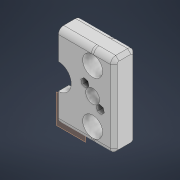
# Autodesk Inventor part: syringe_pump_sledge
Saved by Autodesk Inventor 2022 (Build 260153000, 153)
## iProperties
Created: 2023-04-03
Part Number: syringe_pump_sledge
Material: Generic
Document SubType Name: Modeling
Designer: Jakob Saugbjerg
Density: 1 g/cm^3
Appearance: Default
Author: Jakob Saugbjerg
Autodesk Inventor part; units mm, degrees
ref_plane "YZ Plane" through (0, 0, 0) normal (1, 0, 0) x (0, 1, 0)
ref_plane "XZ Plane" through (0, 0, 0) normal (0, 1, 0) x (-1, 0, 0)
sketch "Sketch1" plane through (0, 0, 0) normal (0, 0, 1) x (1, 0, 0)
  line L0 (0, 0) -> (42, 0)
  line L1 (42, 0) -> (42, 63)
  line L2 (42, 63) -> (0, 63)
  line L3 (0, 63) -> (0, 0)
  dimension "d0" = 42
  dimension "d1" = 63
  constraints: 8 end point, 2 parallel, 1 horizontal, 1 perpendicular
  measures "d0" distance of L2.end L1.end
  measures "d1" distance of L1.end L0.end
extrude "Extrusion1" add sketch "Sketch1" along normal blind 17
sketch "Sketch2" plane through (0, 0, 17) normal (0, 0, 1) x (1, 0, 0)
  line L0 (0, 63) -> (0, 0) projected
  line L1 (0, 31.5) -> (26, 31.5)
  circle A0 centre (26, 31.5) radius 5.25
  dimension "d4" = 26
  dimension "d5" = 10.5
  constraints: 2 end point, 1 centre point, 1 coincident, 1 horizontal, 1 midpoint
  measures "d4" distance of L1.start L1.end
  measures "d5" diameter of A0
extrude "Extrusion2" cut sketch "Sketch2" against normal blind 17
sketch "Sketch4" plane through (0, 0, 17) normal (0, 0, 1) x (1, 0, 0)
  circle A0 centre (26, 31.5) radius 5.25 projected
  line L0 (26, 31.5) -> (26, 51.5)
  line L1 (26, 31.5) -> (26, 11.5)
  circle A1 centre (26, 51.5) radius 7.55
  circle A2 centre (26, 11.5) radius 7.55
  point P0 (0, 0)
  dimension "d14" = 20
  dimension "d15" = 20
  dimension "d16" = 15.1
  dimension "d17" = 15.1
  constraints: 4 end point, 2 centre point, 2 coincident, 2 vertical
  measures "d14" distance of L0.start L0.end
  measures "d15" distance of L0.start L1.end
  measures "d16" diameter of A1
  measures "d17" diameter of A2
extrude "Extrusion4" cut sketch "Sketch4" against normal blind 17 contours A2 | A1
sketch "Sketch5" plane through (0, 0, 17) normal (0, 0, 1) x (1, 0, 0)
  line L0 (0, 63) -> (0, 0) projected
  line L1 (0, 31.5) -> (10, 31.5)
  circle A0 centre (26, 31.5) radius 5.25 projected
  line L2 (26, 31.5) -> (20.1664, 37.3336)
  line L3 (26, 31.5) -> (34.25, 31.5) construction
  line L4 (20.1664, 37.3336) -> (31.8336, 25.6664)
  circle A1 centre (31.8336, 25.6664) radius 1.75
  circle A2 centre (20.1664, 37.3336) radius 1.75
  dimension "d21" = 10
  dimension "d22" = 8.25
  dimension "d23" = 135
  dimension "d24" = 16.5
  dimension "d25" = 3.5
  dimension "d26" = 3.5
  constraints: 8 end point, 2 centre point, 2 coincident, 2 horizontal, 1 equal length, 1 midpoint
  measures "d21" distance of L1.start L1.end
  measures "d22" distance of L2.start L2.end
  measures "d23" angle of L3 L2
  measures "d24" distance of L2.end L4.end
  measures "d25" diameter of A1
  measures "d26" diameter of A2
extrude "Extrusion5" cut sketch "Sketch5" against normal blind 17 contours A1 | A2
ref_plane "Work Plane1" through (0, 0, 7.5) normal (0, 0, 1) x (1, 0, 0)
sketch "Sketch8" plane through (0, 0, 17) normal (0, 0, 1) x (1, 0, 0)
  line L0 (0, 63) -> (0, 0) projected
  circle A0 centre (0, 31.5) radius 9.75
  dimension "d36" = 19.5
  constraints: 1 centre point, 1 midpoint
  measures "d36" diameter of A0
extrude "Extrusion8" cut sketch "Sketch8" against normal blind 10
sketch "Sketch9" plane through (0, 0, 7) normal (0, 0, 1) x (1, 0, 0)
  arc A0 (0, 21.75) -> (0, 41.25) centre (0, 31.5) ccw projected
  circle A1 centre (0, 31.5) radius 12.5
  point P0 (0, 0)
  dimension "d39" = 25
  constraints: 1 centre point, 1 coincident
  measures "d39" diameter of A1
extrude "Extrusion9" [suppressed]
sketch "Sketch10" plane through (0, 0, 0) normal (-1, 0, 0) x (0, 0, 1)
  circle A0 centre (5, 6) radius 1.6
  line L0 (0, 26.25) -> (0, 36.75) projected
  line L1 (0, 31.5) -> (15.0441, 31.5)
  circle A1 centre (5, 57) radius 1.6
  point P0 (0, 0)
  dimension "d42" = 3.2
  constraints: 2 centre point, 2 end point, 1 horizontal, 1 midpoint, 1 symmetric about line, 1 other
  measures "d42" diameter of A0
extrude "Extrusion10" [suppressed]
ref_plane "Work Plane2" through (3, 0, 0) normal (-1, 0, 0) x (0, 0, 1)
sketch "Sketch11" plane through (3, 0, 0) normal (-1, 0, 0) x (0, 0, 1)
  circle A0 centre (5, 6) radius 1.6 projected
  line L0 (5, 6) -> (5, 8.75)
  line L1 (6.5877, 8.75) -> (8.1754, 6)
  line L2 (8.1754, 6) -> (6.5877, 3.25)
  line L3 (6.5877, 3.25) -> (3.4123, 3.25)
  line L4 (3.4123, 3.25) -> (1.8246, 6)
  line L5 (1.8246, 6) -> (3.4123, 8.75)
  line L6 (3.4123, 8.75) -> (6.5877, 8.75)
  circle A1 centre (5, 57) radius 1.6 projected
  line L7 (5, 57) -> (5, 54.25)
  line L8 (3.4123, 54.25) -> (1.8246, 57)
  line L9 (1.8246, 57) -> (3.4123, 59.75)
  line L10 (3.4123, 59.75) -> (6.5877, 59.75)
  line L11 (6.5877, 59.75) -> (8.1754, 57)
  line L12 (8.1754, 57) -> (6.5877, 54.25)
  line L13 (6.5877, 54.25) -> (3.4123, 54.25)
  point P0 (0, 0)
  dimension "d46" = 2.75
  dimension "d47" = 2.75
  constraints: 28 end point, 2 coincident, 2 midpoint, 2 vertical, 26 other
  measures "d46" distance of L0.start L0.end
  measures "d47" distance of L7.start L7.end
extrude "Extrusion11" [suppressed]
sketch "Sketch12" plane through (0, 0, 0) normal (0, 0, -1) x (-1, 0, 0)
  line L0 (-3, 3.25) -> (-5.5, 3.25) projected
  line L1 (-3, 3.25) -> (-5.5, 3.25)
  line L2 (-5.5, 3.25) -> (-5.5, 8.75)
  line L3 (-5.5, 8.75) -> (-3, 8.75)
  line L4 (-3, 8.75) -> (-3, 3.25)
  line L5 (-3, 43.25) -> (-5.5, 43.25) projected
  line L6 (-5.5, 48.75) -> (-5.5, 46) projected
  line L7 (-3, 43.25) -> (-5.5, 43.25)
  line L8 (-5.5, 43.25) -> (-5.5, 48.75)
  line L9 (-5.5, 48.75) -> (-3, 48.75)
  line L10 (-3, 48.75) -> (-3, 43.25)
  point P0 (0, 0)
  constraints: 16 end point, 4 parallel, 2 horizontal, 2 perpendicular
extrude "Extrusion12" [suppressed]
sketch "Sketch13" plane through (0, 0, 0) normal (-1, 0, 0) x (0, 0, 1)
  line L0 (5, 60) -> (9, 60)
  line L1 (9, 60) -> (9, 3)
  line L2 (9, 3) -> (5, 3)
  line L3 (5, 3) -> (5, 60)
  point P0 (0, 0)
  point P1 (5, 31.5)
  dimension "d83" = 4
  constraints: 8 end point, 2 parallel, 1 horizontal, 1 perpendicular
  measures "d83" distance of L1.end L2.end
extrude "Extrusion13" cut sketch "Sketch13" against normal blind 18
fillet "Fillet1" radius 2 2 edges at (0, 3, 7) (0, 60, 7)
sketch "Sketch14" plane through (0, 0, 0) normal (-1, 0, 0) x (0, 0, 1)
  point P0 (0, 0)
sketch "Sketch15" plane through (0, 0, 0) normal (0, 0, -1) x (-1, 0, 0)
  line L0 (0, 21.75) -> (0, 41.25) projected
  line L1 (0, 61.05) -> (0, 53.05)
  line L2 (0, 53.05) -> (-5, 53.05)
  circle A0 centre (-5, 53.05) radius 1.6
  line L3 (0, 0) -> (-42, 0) projected
  line L4 (0, 0) -> (0, 8)
  line L5 (-2, 11.95) -> (-10, 11.95) projected
  line L6 (0, 8) -> (-5, 8)
  circle A1 centre (-5, 8) radius 1.6
  point P0 (0, 9.95)
  dimension "d59" = 8
  dimension "d60" = 5
  dimension "d61" = 3.2
  dimension "d71" = 8
  dimension "d72" = 5
  dimension "d73" = 3.2
  constraints: 8 end point, 3 perpendicular, 2 centre point, 2 coincident, 1 point on line
  measures "d59" distance of L1.start L1.end
  measures "d60" distance of L1.end L2.end
  measures "d61" diameter of A0
  measures "d71" distance of L3.start L4.end
  measures "d72" distance of L4.end L6.end
  measures "d73" diameter of A1
extrude "Extrusion14" [suppressed]
sketch "Sketch17" plane through (0, 0, 17) normal (0, 0, 1) x (1, 0, 0)
  circle A0 centre (5, 53.05) radius 1.6 projected
  line L0 (5, 53.05) -> (5, 50.3)
  line L1 (3.4123, 50.3) -> (1.8246, 53.05)
  line L2 (1.8246, 53.05) -> (3.4123, 55.8)
  line L3 (3.4123, 55.8) -> (6.5877, 55.8)
  line L4 (6.5877, 55.8) -> (8.1754, 53.05)
  line L5 (8.1754, 53.05) -> (6.5877, 50.3)
  line L6 (6.5877, 50.3) -> (3.4123, 50.3)
  circle A1 centre (5, 8) radius 1.6 projected
  line L7 (5, 8) -> (5, 10.75)
  line L8 (6.5877, 10.75) -> (8.1754, 8)
  line L9 (8.1754, 8) -> (6.5877, 5.25)
  line L10 (6.5877, 5.25) -> (3.4123, 5.25)
  line L11 (3.4123, 5.25) -> (1.8246, 8)
  line L12 (1.8246, 8) -> (3.4123, 10.75)
  line L13 (3.4123, 10.75) -> (6.5877, 10.75)
  point P0 (0, 0)
  dimension "d68" = 2.75
  dimension "d76" = 2.75
  constraints: 28 end point, 2 coincident, 2 midpoint, 2 vertical, 26 other
  measures "d68" distance of L0.start L0.end
  measures "d76" distance of L7.start L7.end
extrude "Extrusion15" [suppressed]
sketch "Sketch19" plane through (0, 0, 0) normal (-1, 0, 0) x (0, 0, 1)
  point P0 (0, 0)
sketch "Sketch20" plane through (0, 0, 0) normal (-1, 0, 0) x (0, 0, 1)
  point P0 (0, 0)
fillet "Fillet2" radius 4 4 edges at (21, 0, 0) (21, 63, 0) (21, 63, 17) (21, 0, 17)
sketch "Sketch21" plane through (0, 0, 17) normal (0, 0, 1) x (1, 0, 0)
  circle A0 centre (31.8336, 25.6664) radius 1.75 projected
  line L0 (31.8336, 25.6664) -> (29.8891, 27.6109)
  line L1 (31.8336, 25.6664) -> (34.5836, 25.6664) construction
  circle A1 centre (20.1664, 37.3336) radius 1.75 projected
  line L2 (20.1664, 37.3336) -> (22.1109, 35.3891)
  line L3 (20.9882, 34.2664) -> (17.921, 35.0883)
  line L4 (17.921, 35.0883) -> (17.0991, 38.1555)
  line L5 (17.0991, 38.1555) -> (19.3445, 40.4009)
  line L6 (19.3445, 40.4009) -> (22.4117, 39.579)
  line L7 (22.4117, 39.579) -> (23.2336, 36.5118)
  line L8 (23.2336, 36.5118) -> (20.9882, 34.2664)
  line L9 (31.0118, 28.7336) -> (34.079, 27.9117)
  line L10 (34.079, 27.9117) -> (34.9009, 24.8445)
  line L11 (34.9009, 24.8445) -> (32.6555, 22.5991)
  line L12 (32.6555, 22.5991) -> (29.5883, 23.421)
  line L13 (29.5883, 23.421) -> (28.7664, 26.4882)
  line L14 (28.7664, 26.4882) -> (31.0118, 28.7336)
  point P0 (0, 0)
  dimension "d78" = 2.75
  dimension "d79" = 135
  dimension "d80" = 2.75
  constraints: 30 end point, 2 coincident, 2 midpoint, 1 equal length, 1 horizontal, 26 other
  measures "d78" distance of L0.start L0.end
  measures "d79" angle of L1 L0
  measures "d80" distance of L2.start L2.end
extrude "Extrusion16" cut sketch "Sketch21" against normal blind 5
chamfer "Chamfer1" distance 2.5 angle 45 8 edges at (42, 31.5, 17) (42, 61.8284, 15.8284) (42, 63, 8.5) (42, 61.8284, 1.1716) (42, 31.5, 0) (42, 1.1716, 1.1716) (42, 0, 8.5) (42, 1.1716, 15.8284)
body "Solid1"
